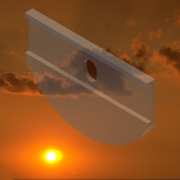
# Autodesk Inventor part: C11_ZP_middle wheel plate
Saved by Autodesk Inventor 2015 SP1 (Build 190203100, 203)
## iProperties
Created: 2016-01-16
Part Number: C11_ZP_middle wheel plate
Material: Generic
Document SubType Name: Modeling
Designer: Administrator
Density: 1 g/cm^3
Appearance: Polycarbonate - Clear
Author: Administrator
Autodesk Inventor part; units mm, degrees
ref_plane "YZ Plane" through (0, 0, 0) normal (1, 0, 0) x (0, 1, 0)
ref_plane "XZ Plane" through (0, 0, 0) normal (0, 1, 0) x (-1, 0, 0)
ref_plane "XY Plane" through (0, 0, 0) normal (0, 0, 1) x (1, 0, 0)
sketch "Sketch1" plane through (0, 0, 0) normal (0, 0, 1) x (1, 0, 0)
  line L0 (0, 0) -> (0, 63.5)
  line L1 (0, 63.5) -> (203.2, 63.5)
  line L2 (203.2, 63.5) -> (203.2, 0)
  line L3 (0, 0) -> (203.2, 0)
  dimension "d0" = 63.5
  dimension "d1" = 203.2
  constraints: 8 end point, 2 perpendicular, 1 horizontal, 1 vertical
  measures "d0" distance of L0.start L0.end
  measures "d1" distance of L0.end L1.end
extrude "Extrusion1" add sketch "Sketch1" along normal blind 12.7
sketch "Sketch2" plane through (0, 0, 12.7) normal (0, 0, 1) x (1, 0, 0)
  line L0 (0, 63.5) -> (0, 0) projected
  line L1 (203.2, 0) -> (203.2, 63.5) projected
  line L2 (0, 57.15) -> (203.2, 57.15)
  line L3 (203.2, 57.15) -> (203.2, 6.35)
  line L4 (203.2, 6.35) -> (0, 6.35)
  line L5 (0, 6.35) -> (0, 57.15)
  line L6 (0, 63.5) -> (203.2, 63.5) projected
  line L7 (203.2, 0) -> (0, 0) projected
  dimension "d4" = 6.35
  dimension "d5" = 6.35
  constraints: 8 end point, 2 parallel, 2 point on line, 1 horizontal, 1 perpendicular
  measures "d4" distance between parallel lines of L6 L2
  measures "d5" distance between parallel lines of L7 L4
extrude "Extrusion2" cut sketch "Sketch2" against normal blind 6.35 contours L2 L1 L4 L0
sketch "Sketch3" plane through (0, 0, 6.35) normal (0, 0, 1) x (1, 0, 0)
  arc A0 (0, 0) -> (203.2, 0) centre (101.6, 50.8) ccw
  line L0 (0, 0) -> (203.2, 0) projected
  dimension "d8" = 50.8
  constraints: 2 point on circle, 1 centre point
  measures "d8" distance from line of A0.centre L0
extrude "Extrusion3" add sketch "Sketch3" along normal mid plane 12.7
sketch "Sketch4" plane through (0, 0, 6.35) normal (0, 0, 1) x (1, 0, 0)
  circle A0 centre (101.6, 31.75) radius 11.1125
  circle A1 centre (101.6, 24.13) radius 11.1125
  line L0 (203.2, 57.15) -> (203.2, 6.35) projected
  line L1 (0, 57.15) -> (203.2, 57.15) projected
  line L2 (90.4875, 31.75) -> (90.4875, 24.13)
  line L3 (112.7125, 31.75) -> (112.7125, 24.13)
  point P0 (0, 0)
  dimension "d11" = 101.6
  dimension "d12" = 101.6
  dimension "d13" = 22.225
  dimension "d14" = 7.62
  dimension "d15" = 22.225
  dimension "d16" = 25.4
  constraints: 4 end point, 4 point on circle, 2 centre point, 2 tangent, 2 vertical
  measures "d11" distance from line of L0 A0.centre
  measures "d12" distance from line of L0 A1.centre
  measures "d13" diameter of A0
  measures "d14" distance of A1.centre A0.centre
  measures "d15" diameter of A1
  measures "d16" distance from line of L1 A0.centre
extrude "Extrusion4" cut sketch "Sketch4" against normal blind 12.7
body "Solid1"
